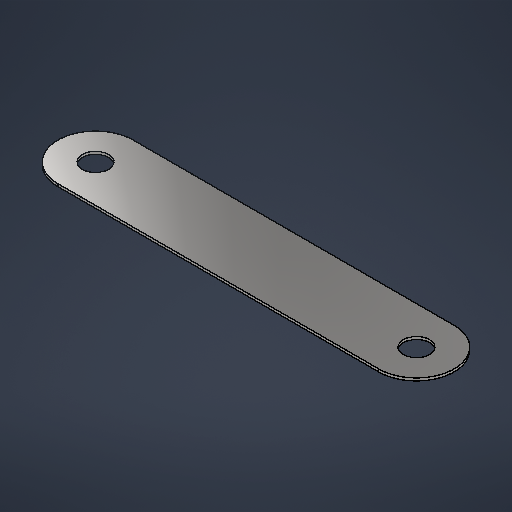
# Autodesk Inventor part: Part16.5mm
Saved by Autodesk Inventor 2026 (Build 300175050, 175E)
## iProperties
Created: 2025-07-21
Part Number: Part16.5mm
Material: Steel, Carbon
Document SubType Name: Sheet Metal
Designer: Joshua Eah
Density: 7.85 g/cm^3
Sheet Metal Rule: 0.4mm Spring Steel
Appearance: Semi-Polished
Author: Joshua Eah
Autodesk Inventor part; units mm, degrees
ref_plane "YZ Plane" through (0, 0, 0) normal (1, 0, 0) x (0, 1, 0)
ref_plane "XZ Plane" through (0, 0, 0) normal (0, 1, 0) x (-1, 0, 0)
ref_plane "XY Plane" through (0, 0, 0) normal (0, 0, 1) x (1, 0, 0)
sketch "Sketch1" plane through (0, 0, 0) normal (0, 1, 0) x (-1, 0, 0)
  line L0 (0, 0) -> (-68.3, 0) construction
  line L1 (-6.5, 6.5) -> (-61.8, 6.5)
  line L2 (-61.8, -6.5) -> (-6.5, -6.5)
  arc A0 (-6.5, -6.5) -> (-6.5, 6.5) centre (-6.5, 0) ccw
  arc A1 (-61.8, 6.5) -> (-61.8, -6.5) centre (-61.8, 0) ccw
  line L3 (-23.9184, -1.1237) -> (-43.8581, -1.1237) construction
  line L4 (-43.8581, -1.1237) -> (-43.8581, 0.6417) construction
  line L5 (-43.8581, 0.6417) -> (-23.9184, 0.6417) construction
  line L6 (-23.9184, 0.6417) -> (-23.9184, -1.1237) construction
  line L7 (-34.15, -6.5) -> (-34.15, 6.5) construction
  point P0 (-34.15, 0)
  dimension "MinimumRemnant" = 0.9
  dimension "d21" = 68.3
  dimension "d22" = 13
  constraints: 10 end point, 6 point on circle, 4 tangent, 3 midpoint, 2 centre point, 2 point on line, 1 horizontal, 1 parallel, 2 other
  measures "d21" distance of L0.start L0.end
  measures "d22" diameter of A1
extrude "Plate2" add sketch "Sketch1" against normal blind 0.45
hole "Hole2" at (6.5, 0, 0) at (61.8, 0, 0) direction (0, -1, 0) diameter 4.4958 end through all clearance for "Socket Head Cap Screw" size "M4" standard "Ansi Metric M Profile"
equation "\"MinimumRemnant\" = 2 * Thickness"
equation "\"d29\" = Thickness"
equation "\"d23\" = Thickness"
equation "\"BendRadius\" = Thickness"
equation "\"BendReliefWidth\" = Thickness"
equation "\"BendReliefDepth\" = 0.5 * Thickness"
equation "\"CornerReliefSize\" = 4 * Thickness"
equation "\"TransitionRadius\" = BendRadius"
equation "\"JacobiRadiusSize\" = BendRadius"
equation "\"GapSize\" = Thickness"
equation "\"radius\" = 6"
equation "\"Thickness\" = 0.45"
body "Solid2"
